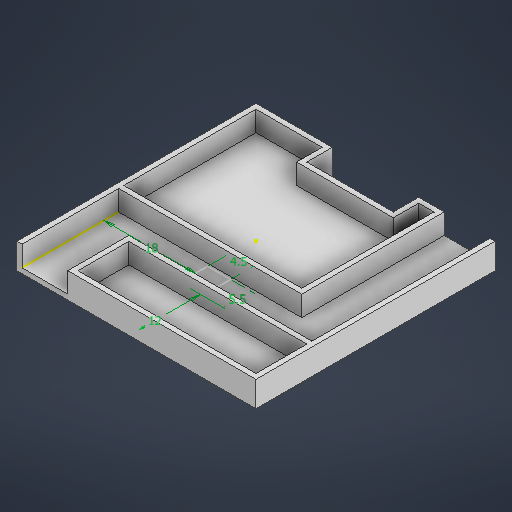
# Autodesk Inventor part: particle_sensor_case_top
Saved by Autodesk Inventor 2027 (Build 310192060, 192F)
## iProperties
Created: 2026-06-05
Part Number: particle_sensor_case_top
Material: Generic
Document SubType Name: Modeling
Designer: cmitchel
Density: 1 g/cm^3
Appearance: Default
Author: cmitchel
Autodesk Inventor part; units mm, degrees
ref_plane "YZ Plane" through (0, 0, 0) normal (1, 0, 0) x (0, 1, 0)
ref_plane "XZ Plane" through (0, 0, 0) normal (0, 1, 0) x (-1, 0, 0)
ref_plane "XY Plane" through (0, 0, 0) normal (0, 0, 1) x (1, 0, 0)
sketch "Sketch1" plane through (0, 0, 0) normal (0, 1, 0) x (-1, 0, 0)
  point P0 (0, 0)
sketch "Sketch2" plane through (0, 0, 0) normal (0, 1, 0) x (-1, 0, 0)
  line L0 (23.5, 23.5) -> (-23.5, 23.5)
  line L1 (-23.5, 23.5) -> (-23.5, -23.5)
  line L2 (23.5, -23.5) -> (23.5, 23.5)
  line L3 (8.5, -18.5) -> (-8.5, -18.5)
  line L4 (-8.5, -23.5) -> (-8.5, -18.5)
  line L5 (8.5, -18.5) -> (8.5, -23.5)
  line L6 (-23.5, -23.5) -> (-8.5, -23.5)
  line L7 (8.5, -23.5) -> (23.5, -23.5)
  point P0 (0, 0)
  dimension "d4" = 47
  dimension "d5" = 47
  dimension "d7" = 23.5
  dimension "d41" = 15
  dimension "d42" = 15
  constraints: 16 end point, 5 perpendicular, 3 parallel, 1 horizontal
  measures "d4" distance of L2.start L1.end
  measures "d5" distance of L2.start L2.end
  measures "d7" distance from line of point (0, 0) L2
  measures "d41" distance between parallel lines of L1 L4
  measures "d42" distance between parallel lines of L2 L5
extrude "Extrusion1" add sketch "Sketch2" along normal blind 5
sketch "Sketch3" plane through (0, 5, 0) normal (0, 1, 0) x (1, 0, 0)
  point P0 (0, 0)
sketch "Sketch4" plane through (0, 5, 0) normal (0, 1, 0) x (1, 0, 0)
  line L0 (22.5, -22.5) -> (22.5, 22.5)
  line L1 (-22.5, 22.5) -> (-22.5, -31.5)
  line L2 (22.5, 22.5) -> (13.5356, 22.5)
  line L3 (22.5, 11) -> (22.5, 22.5)
  line L4 (13.5, -4.5) -> (-22.5, -4.5)
  line L5 (-22.5, -4.5) -> (-22.5, -23.5)
  line L6 (-23.5, 23.5) -> (-23.5, -23.5) projected
  line L7 (-22.5, -23.5) -> (-13.5, -23.5)
  line L8 (-13.5, -23.5) -> (-13.5, -11.5)
  line L9 (-13.5, -11.5) -> (22.5, -11.5)
  line L10 (13.5, -4.5) -> (13.5, 23.5)
  line L11 (13.5, 23.5) -> (22.5, 23.5)
  line L12 (22.5, 23.5) -> (22.5, -11.5)
  line L13 (22.5, -22.5) -> (-12.5, -22.5)
  line L14 (-12.5, -22.5) -> (-12.5, -12.5)
  line L15 (-12.5, -12.5) -> (22.5, -12.5)
  line L16 (22.5, -12.5) -> (22.5, -22.5)
  line L17 (12.5, 22.5) -> (12.5, -3.5)
  line L18 (12.5, -3.5) -> (-22.5, -3.5)
  line L19 (-22.5, -3.5) -> (-22.5, 22.5)
  line L20 (-9.5, 22.5) -> (-9.5, 17.5)
  line L21 (-9.5, 17.5) -> (9.5, 17.5)
  line L22 (9.5, 17.5) -> (9.5, 22.5)
  line L23 (-8.5, 18.5) -> (-8.5, 23.5) projected
  line L24 (8.5, 23.5) -> (8.5, 18.5) projected
  line L25 (22.5, 22.5) -> (8.5, 22.5)
  line L26 (-8.5, 22.5) -> (-22.5, 22.5)
  line L27 (-22.5, 22.5) -> (-8.5, 22.5)
  line L28 (8.5, 22.5) -> (12.5, 22.5)
  line L29 (-5, -3.5) -> (-20.0496, -3.5)
  line L30 (-20.0496, -3.5) -> (-20.0496, 2.4851)
  line L31 (-20.0496, 2.4851) -> (-5, 2.4851)
  line L32 (-5, 2.4851) -> (-5, -3.5)
  line L33 (-23.5, -23.5) -> (23.5, -23.5) projected
  line L34 (23.5, 23.5) -> (8.5, 23.5) projected
  point P0 (0, 0)
  point P1 (22.5, 22.5)
  point P2 (22.5, -12.5)
  point P3 (-22.5, -3.5)
  point P4 (-9.5, 20)
  point P5 (8.5, 21)
  point P6 (12.5, 22.5)
  point P7 (13.5, 22.5)
  point P8 (9.5, 22.5)
  point P9 (22.5, 22.5)
  point P10 (10.5, 22.5)
  dimension "d10" = 45
  dimension "d13" = 22.5
  dimension "d33" = 9
  dimension "d36" = 1
  dimension "d38" = 1
  dimension "d39" = 1
  dimension "d43" = 5
  dimension "d44" = 1
  dimension "d45" = 1
  dimension "d50" = 1
  dimension "d51" = 11
  dimension "d52" = 18
  dimension "d53" = 1
  dimension "d54" = 1
  constraints: 60 end point, 14 perpendicular, 9 parallel, 5 horizontal, 5 midpoint, 5 point on line, 1 collinear
  measures "d10" distance between parallel lines of L0 L1
  measures "d13" distance from line of point (0, 0) L1
  measures "d33" distance of L10.end L11.end
  measures "d36" distance between parallel lines of L9 L15
  measures "d38" distance between parallel lines of L4 L18
  measures "d39" distance between parallel lines of L10 L17
  measures "d43" distance of L20.start L20.end
  measures "d44" distance from line of L23 point (-9.5, 20)
  measures "d45" distance from line of point (8.5, 21) L22
  measures "d50" distance between parallel lines of L8 L14
  measures "d51" distance between parallel lines of L9 L13
  measures "d52" distance between parallel lines of L4 L13
  measures "d53" distance between parallel lines of L33 L13
  measures "d54" distance from line of point (10.5, 22.5) L34
extrude "Extrusion5" cut sketch "Sketch4" against normal blind 4 contours L13 L14 L15 L0 | L9 L8 L7 L1 L4 L10 L25 L2 L0 | L2 L25 L10 L11 L12 | L17 L18 L32 L31 L30 L1 L26 L20 L21 L22 L25 | L30 L31 L32 L18
sketch "PD placement" plane through (0, 1, 0) normal (0, 1, 0) x (1, 0, 0)
  line L0 (-4.5, -10.5) -> (0, -10.5)
  line L1 (0, -10.5) -> (0, -5)
  line L2 (0, -5) -> (-4.5, -5)
  line L3 (-4.5, -5) -> (-4.5, -10.5)
  line L4 (22.5, -22.5) -> (-12.5, -22.5) projected
  line L5 (22.5, 23.5) -> (22.5, -11.5) projected
  line L6 (-22.5, -23.5) -> (-22.5, -4.5) projected
  point P0 (0, 0)
  dimension "d55" = 4.5
  dimension "d56" = 5.5
  dimension "d57" = 12
  dimension "d59" = 18
  constraints: 8 end point, 2 parallel, 1 horizontal, 1 perpendicular
  measures "d55" distance of L2.end L1.end
  measures "d56" distance of L0.end L1.end
  measures "d57" distance between parallel lines of L4 L0
  measures "d59" distance between parallel lines of L6 L3
body "Solid1"
